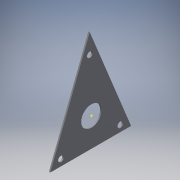
# Autodesk Inventor part: fixação KS traseiro
Saved by Autodesk Inventor 2019 (Build 230136000, 136)
## iProperties
Created: 2020-05-17
Part Number: fixação KS traseiro
Material: Genérico
Document SubType Name: Modeling
Designer: eliane
Density: 1 g/cm^3
Appearance: Padrão
Categories: <MemberInstance><Categories><Category DisplayName="" Mnemonic="CABLEANDHARNESS" InternalName="e4a7e005-5e42-4d16-b293-125e7f0d0512"><Category DisplayName="" Mnemonic="CONNECTORS" InternalName="6f634eba-a678-4820-a31d-2c2d5ee6728e"><CategoryParameter DisplayName="" Mnemonic="REFDES" InternalName="c3740e8c-60ab-4d5d-8584-52b73222f2f0"/><Category DisplayName="" Mnemonic="DISCRETEWIRE" InternalName="9a3407de-09b2-4cdb-8c40-9708d5144a28"/></Category></Category></Categories><FamilyTemplate><FamilyTemplateParameters></FamilyTemplateParameters></FamilyTemplate><CategoryParameterMap><ParamToTemplateMap><ParamToTemplate CategoryParameter="//CategoryParameter[@InternalName='c3740e8c-60ab-4d5d-8584-52b73222f2f0']" ConstantValue=""/></ParamToTemplateMap></CategoryParameterMap></MemberInstance>
Author: eliane
Autodesk Inventor part; units mm, degrees
ref_plane "YZ Plane" through (0, 0, 0) normal (1, 0, 0) x (0, 1, 0)
ref_plane "XZ Plane" through (0, 0, 0) normal (0, 1, 0) x (-1, 0, 0)
ref_plane "XY Plane" through (0, 0, 0) normal (0, 0, 1) x (1, 0, 0)
sketch "Esboço1" plane through (0, 0, 0) normal (1, 0, 0) x (0, 1, 0)
  line L0 (0, 0) -> (0, 43) construction
  line L1 (0, 0) -> (0, -43) construction
  line L2 (0, 0) -> (-40, 0) construction
  line L3 (-40, -43) -> (-40, 44.381)
  line L4 (-40, 0) -> (66, 0) construction
  line L5 (-40, -43) -> (70.202, 1.7046)
  line L6 (70.202, 1.7046) -> (-40, 44.381)
  circle A0 centre (-9.265, 0) radius 11
  line L7 (-326.6157, 155.3746) -> (103.2483, -11.0928)
  dimension "d1" = 43
  dimension "d2" = 43
  dimension "d3" = 40
  dimension "d4" = 106
  dimension "d5" = 22
  constraints: 16 end point, 3 point on line, 3 vertical, 1 centre point, 1 coincident, 3 other
  measures "d1" distance of L0.start L0.end
  measures "d2" distance of L0.start L1.end
  measures "d3" distance of L0.start L2.end
  measures "d4" distance of L4.end L2.end
  measures "d5" diameter of A0
extrude "Extrusão1" add sketch "Esboço1" along normal blind 1.5
sketch "Esboço2" plane through (0, 0, 0) normal (-1, 0, 0) x (0, 0, 1)
  circle A0 centre (1.7046, 49.0262) radius 3 projected
  circle A1 centre (-31.3462, -33.0501) radius 3 projected
  circle A2 centre (32.9237, -33.0501) radius 3 projected
  point P0 (0, 0)
extrude "Extrusão2" cut sketch "Esboço2" against normal blind 2
sketch "Esboço3" plane through (1.5, 0, 0) normal (1, 0, 0) x (0, 0, -1)
  circle A0 centre (0, -9.265) radius 11 projected
